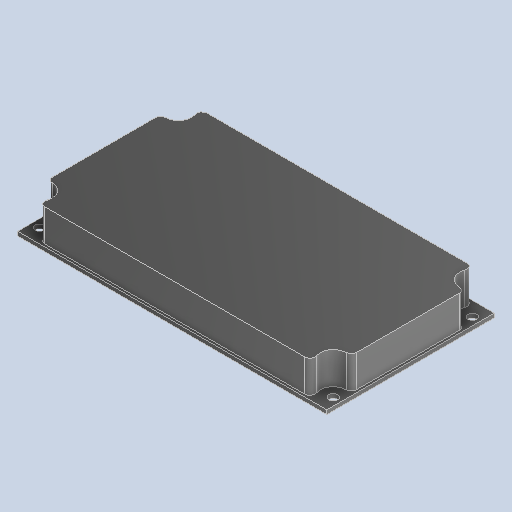
# Autodesk Inventor part: SUSTAINA-CORE-BOARD
Saved by Autodesk Inventor 2024.2 (Build 282272000, 272)
## iProperties
Created: 2024-01-24
Part Number: SUSTAINA-CORE-BOARD
Material: Acetal Resin, Black
Document SubType Name: Modeling
Designer: Masato Kubotera
Density: 1.425 g/cm^3
Appearance: Smooth - Black
Mass: 222.562 g
Surface Area: 231.578 cm^2
Volume: 156.184 cm^3
Author: Masato Kubotera
Autodesk Inventor part; units mm, degrees
ref_plane "YZ Plane" through (0, 0, 0) normal (1, 0, 0) x (0, 1, 0)
ref_plane "XZ Plane" through (0, 0, 0) normal (0, 1, 0) x (-1, 0, 0)
ref_plane "XY Plane" through (0, 0, 0) normal (0, 0, 1) x (1, 0, 0)
sketch "Sketch1" plane through (0, 0, 0) normal (0, 0, 1) x (1, 0, 0)
  line L0 (32.5, 60) -> (-32.5, 60)
  line L1 (-32.5, 60) -> (-32.5, -60)
  line L2 (-32.5, -60) -> (32.5, -60)
  line L3 (32.5, -60) -> (32.5, 60)
  line L4 (32.5, 60) -> (-32.5, -60) construction
  line L5 (-32.5, 60) -> (32.5, -60) construction
  line L6 (-27, 57) -> (27, 57) construction
  line L7 (27, 57) -> (27, -57) construction
  line L8 (27, -57) -> (-27, -57) construction
  line L9 (-27, -57) -> (-27, 57) construction
  line L10 (-27, 57) -> (27, -57) construction
  line L11 (27, 57) -> (-27, -57) construction
  arc A0 (22.4174, 59) -> (31.5, 54.8206) centre (27, 57) ccw
  line L12 (31.5, 54.8206) -> (31.5, -54.8206)
  line L13 (22.4174, 59) -> (-22.4174, 59)
  line L14 (32.5, 0) -> (-32.5, 0) construction
  line L15 (0, 60) -> (0, -60) construction
  arc A1 (31.5, -54.8206) -> (22.4174, -59) centre (27, -57) ccw
  line L16 (22.4174, -59) -> (-22.4174, -59)
  arc A2 (-31.5, 54.8206) -> (-22.4174, 59) centre (-27, 57) ccw
  line L17 (-31.5, 54.8206) -> (-31.5, -54.8206)
  arc A3 (-22.4174, -59) -> (-31.5, -54.8206) centre (-27, -57) ccw
  point P0 (0, 0)
  dimension "d0" = 65
  dimension "d1" = 120
  dimension "d2" = 5.5
  dimension "d3" = 3
  dimension "d4" = 1
  dimension "d5" = 1
  dimension "d6" = 5
  constraints: 36 end point, 10 symmetric about line, 8 midpoint, 8 point on circle, 5 coincident, 4 centre point, 4 parallel, 3 horizontal, 2 perpendicular, 1 vertical, 3 other
  measures "d0" distance of L2.end L1.end
  measures "d1" distance of L1.end L0.end
  measures "d2" distance between parallel lines of L7 L3
  measures "d3" distance between parallel lines of L0 L6
  measures "d4" distance between parallel lines of L12 L3
  measures "d5" distance between parallel lines of L0 L13
  measures "d6" radius of A0
extrude "Extrusion1" add sketch "Sketch1" along normal blind 1.6 contours L3 L2 L1 L0 | A0 L12 A1 L16 A3 L17 A2 L13
extrude "Extrusion2" add sketch "Sketch1" along normal blind 14.1 contours A0 L12 A1 L16 A3 L17 A2 L13
hole "Hole1" at (27, 57, 0) at (-27, 57, 0) at (-27, -57, 0) at (27, -57, 0) direction (0, 0, 1) diameter 3.5 end through all
fillet "Fillet1" radius 2 8 edges at (-22.4174, 59, 7.85) (-31.5, 54.8206, 7.85) (22.4174, 59, 7.85) (31.5, 54.8206, 7.85) (31.5, -54.8206, 7.85) (22.4174, -59, 7.85) (-22.4174, -59, 7.85) (-31.5, -54.8206, 7.85)
equation "\"d5\" = d4"
body "Solid1"
